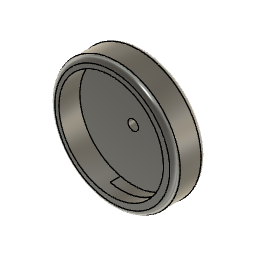
Rengas v3 (Autodesk Fusion 360 design; units mm, degrees)
Autodesk Fusion 360 part; units mm, degrees
cylinder "CylinderPrimitive2" add diameter 60 height 15 placed x (1, 0, 0) y (0, 0, -1) z (0, 1, 0) at (0, 0, 0)
hole "Hole2" at (-0.2955, 0, 0.3154) direction (0, 1, 0) diameter 5 depth 15 tip angle 180
delete_face "DeleteFace1" 1 faces at (-0.0466, 5, -2.1722)
fillet "Fillet1" radius 2.5 2 edges at (-27.9698, 15, 10.8485) (-27.9698, 0, -10.8485)
shell "Shell1" thickness 5 removed faces 0 bodies 1
hole "Hole3" at (-0.5581, 0, 0.1324) direction (0, 1, 0) diameter 50 depth 10 tip angle 180
hole "Hole4" at (0, 10, 0) direction (0, 1, 0) diameter 5 depth 5 tip angle 180
